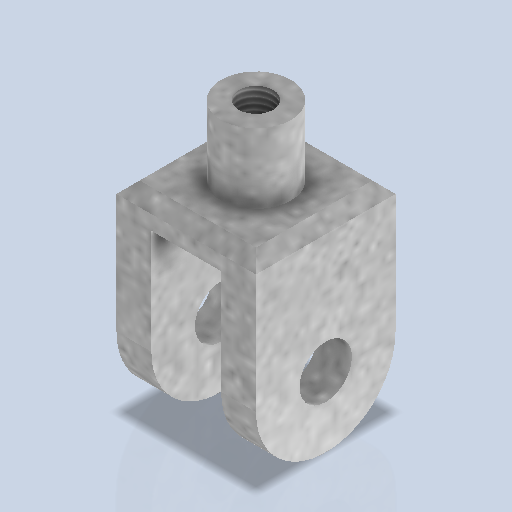
# Autodesk Inventor part: top_cylinder
Saved by Autodesk Inventor 2024.2 (Build 282272000, 272)
## iProperties
Created: 2024-05-05
Part Number: top_cylinder
Material: Glasfaserbeton
Document SubType Name: Modeling
Designer: Fabri
Density: 1.7 g/cm^3
Appearance: Flach - Poliert Grau
Author: Fabri
Autodesk Inventor part; units mm, degrees
note: some values were not read from the file. Chosen so that the rebuilt part matches the saved one: direction of "Bohrung1".
ref_plane "YZ Plane" through (0, 0, 0) normal (1, 0, 0) x (0, 1, 0)
ref_plane "XZ Plane" through (0, 0, 0) normal (0, 1, 0) x (-1, 0, 0)
ref_plane "XY Plane" through (0, 0, 0) normal (0, 0, 1) x (1, 0, 0)
sketch "Skizze1" plane through (0, 0, 0) normal (0, 1, 0) x (-1, 0, 0)
  line L0 (0, 0) -> (24, 0)
  line L1 (24, 0) -> (24, -34.5)
  line L2 (24, -34.5) -> (18, -34.5)
  line L3 (18, -34.5) -> (18, -4.5)
  line L4 (18, -4.5) -> (6, -4.5)
  line L5 (6, -4.5) -> (6, -34.5)
  line L6 (6, -34.5) -> (0, -34.5)
  line L7 (0, -34.5) -> (0, 0)
  dimension "d0" = 6
  dimension "d1" = 6
  dimension "d2" = 12
  dimension "d3" = 30
  dimension "d4" = 4.5
  constraints: 16 end point, 4 perpendicular, 2 parallel, 2 point on line, 1 horizontal
  measures "d0" distance between parallel lines of L7 L5
  measures "d1" distance between parallel lines of L3 L1
  measures "d2" distance between parallel lines of L5 L3
  measures "d3" distance between parallel lines of L6 L4
  measures "d4" distance between parallel lines of L4 L0
extrude "Extrusion1" add sketch "Skizze1" along normal blind 24
fillet "Rundung1" radius 12 2 edges at (-3, 24, -34.5) (-3, 0, -34.5)
fillet "Rundung2" radius 12 2 edges at (-21, 0, -34.5) (-21, 24, -34.5)
sketch "Skizze2" plane through (0, 0, 0) normal (1, 0, 0) x (0, 0, -1)
  arc A0 (22.5, 0) -> (22.5, 24) centre (22.5, 12) ccw projected
  point P0 (0, 0)
  constraints: 1 coincident
hole "Bohrung1" at (0, 12, -22.5) direction (-1, 0, 0) diameter 9 depth 24
chamfer "Fasen1" distance 2 angle 45 4 edges at (-12, 24, 0) (0, 12, 0) (-12, 0, 0) (-24, 12, 0)
sketch "Skizze3" plane through (-22, 2, 0) normal (0, 0, 1) x (1, 0, 0)
  circle A0 centre (10, 10) radius 6
  line L0 (-2, 22) -> (-2, -2) projected
  line L1 (0, 20) -> (20, 20) projected
  point P0 (22, -2)
  point P1 (-2, 10)
  point P2 (10, 20)
  dimension "d19" = 12
  constraints: 2 midpoint, 1 centre point, 1 horizontal alignment, 1 vertical alignment
  measures "d19" diameter of A0
extrude "Extrusion2" add sketch "Skizze3" along normal blind 12
sketch "Skizze4" plane through (-12, 12, 12) normal (0, 0, 1) x (1, 0, 0)
  circle A0 centre (0, 0) radius 6 projected
  point P0 (12, -12)
  constraints: 1 coincident
hole "Bohrung2" at (-12, 12, 12) direction (0, 0, -1) diameter 5.9175 depth 16.5 tip angle 118 thread size "M7x1" class "6H" standard "ISO Metric profile"
